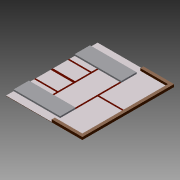
# Autodesk Inventor part: Ball Field
Saved by Autodesk Inventor 2015 (Build 190159000, 159)
## iProperties
Created: 2016-11-29
Part Number: Ball Field
Material: Generic
Document SubType Name: Modeling
Designer: Simms
Density: 1 g/cm^3
Appearance: Default
Author: Simms
Autodesk Inventor part; units mm, degrees
ref_plane "YZ Plane" through (0, 0, 0) normal (1, 0, 0) x (0, 1, 0)
ref_plane "XZ Plane" through (0, 0, 0) normal (0, 1, 0) x (-1, 0, 0)
ref_plane "XY Plane" through (0, 0, 0) normal (0, 0, 1) x (1, 0, 0)
sketch "Sketch1" plane through (0, 0, 0) normal (0, 1, 0) x (-1, 0, 0)
  line L0 (0, 381) -> (-635, 381)
  line L1 (-635, 381) -> (-635, -381)
  line L2 (-635, -381) -> (0, -381)
  line L3 (0, 0) -> (-635, -381) construction
  line L4 (-635, 381) -> (0, 0) construction
  line L5 (0, 381) -> (0, -381)
  point P0 (0, 0)
  dimension "d1" = 762
  constraints: 12 end point, 2 point on line, 1 horizontal, 1 midpoint, 1 parallel, 1 perpendicular
  measures "d1" distance of L1.end L0.end
extrude "Extrusion1" add sketch "Sketch1" along normal blind 2.54
sketch "Sketch2" plane through (0, 2.54, 0) normal (0, 1, 0) x (1, 0, 0)
  line L0 (0, -381) -> (635, -381) projected
  line L1 (635, -381) -> (635, 381) projected
  line L2 (635, 381) -> (0, 381) projected
  line L3 (609.6, -355.6) -> (381, -355.6)
  line L4 (381, 355.6) -> (609.6, 355.6)
  line L5 (609.6, 355.6) -> (609.6, -355.6)
  line L6 (381, -381) -> (381, -355.6)
  line L7 (381, 355.6) -> (381, 381)
  line L8 (0, 381) -> (0, -381) projected
  line L9 (381, -355.6) -> (381, 355.6) construction
  line L10 (374.65, 190.5) -> (374.65, -190.5)
  line L11 (609.6, 6.35) -> (609.6, -6.35)
  line L12 (609.6, -6.35) -> (387.35, -6.35)
  line L13 (387.35, -190.5) -> (387.35, -6.35)
  line L14 (387.35, 6.35) -> (387.35, 190.5)
  line L15 (387.35, 6.35) -> (609.6, 6.35)
  line L16 (0, -190.5) -> (0, -317.5)
  line L17 (0, -317.5) -> (387.35, -317.5)
  line L18 (387.35, -317.5) -> (387.35, -190.5)
  line L19 (374.65, -190.5) -> (0, -190.5)
  line L20 (0, 0) -> (635, 0) construction
  line L21 (0, 190.5) -> (0, 317.5)
  line L22 (0, 317.5) -> (387.35, 317.5)
  line L23 (387.35, 317.5) -> (387.35, 190.5)
  line L24 (374.65, 190.5) -> (0, 190.5)
  line L25 (196.85, 190.5) -> (196.85, -190.5)
  line L26 (374.65, -190.5) -> (387.35, -190.5)
  line L27 (374.65, 190.5) -> (387.35, 190.5)
  line L28 (0, 0) -> (190.5, 0) construction
  line L29 (184.15, -9.525) -> (0, -9.525)
  line L30 (0, -9.525) -> (0, 9.525)
  line L31 (0, 9.525) -> (184.15, 9.525)
  line L32 (0, 133.35) -> (184.15, 133.35)
  line L33 (0, 146.05) -> (0, 133.35)
  line L34 (184.15, 146.05) -> (0, 146.05)
  line L35 (184.15, 9.525) -> (184.15, 133.35)
  line L36 (184.15, 146.05) -> (184.15, 190.5)
  line L37 (0, -133.35) -> (184.15, -133.35)
  line L38 (0, -146.05) -> (0, -133.35)
  line L39 (184.15, -146.05) -> (0, -146.05)
  line L40 (184.15, -190.5) -> (184.15, -146.05)
  line L41 (184.15, -133.35) -> (184.15, -9.525)
  line L42 (381, -381) -> (635, -381)
  line L43 (635, -381) -> (635, 381)
  line L44 (635, 381) -> (381, 381)
  line L45 (635, 381) -> (0, 381) projected
  point P0 (495.3, 0)
  point P1 (95.25, 0)
  point P2 (95.25, 88.9)
  dimension "d4" = 25.4
  dimension "d5" = 254
  dimension "d8" = 12.7
  dimension "d11" = 127
  dimension "d16" = 19.05
  dimension "d19" = 63.5
  dimension "d21" = 44.45
  dimension "d22" = 12.7
  dimension "d23" = 374.65
  constraints: 83 end point, 11 parallel, 7 horizontal, 7 symmetric about line, 4 point on line, 3 collinear, 3 perpendicular, 2 midpoint, 2 vertical
  measures "d4" distance between parallel lines of L0 L3
  measures "d5" distance from line of L3.end L1
  measures "d8" distance of L10.start L14.end
  measures "d11" distance of L16.end L16.start
  measures "d16" distance of L29.end L30.end
  measures "d19" distance between parallel lines of L17 L0
  measures "d21" distance between parallel lines of L24 L34
  measures "d22" distance between parallel lines of L15 L12
  measures "d23" distance between parallel lines of L12 L0
extrude "Extrusion2" add sketch "Sketch2" along normal blind 12.7 contours L8 L19 L26 L18 L17 | L24 L8 L22 L23 L27
extrude "Extrusion3" add sketch "Sketch2" along normal blind 19.05 contours L6 L3 L5 L4 L7 L2 L1 L0
extrude "Extrusion4" add sketch "Sketch2" along normal blind 0.254 contours L8 L37 L41 L29 L31 L35 L32 L34 L36 L24 L25 L19 L40 L39 | L26 L10 L27 L14 L15 L5 L12 L13
body "Solid1"
